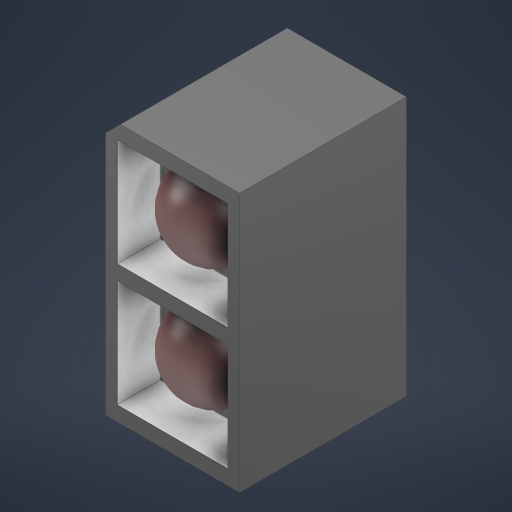
# Autodesk Inventor part: LBR127HLD
Saved by Autodesk Inventor 2023 (Build 270158000, 158)
## iProperties
Created: 2022-09-02
Part Number: LBR127HLD
Material: 一般
Document SubType Name: Modeling
Designer: neko2
Density: 1 g/cm^3
Appearance: 既定
Author: neko2
Autodesk Inventor part; units mm, degrees
ref_plane "YZ Plane" through (0, 0, 0) normal (1, 0, 0) x (0, 1, 0)
ref_plane "XZ Plane" through (0, 0, 0) normal (0, 1, 0) x (-1, 0, 0)
ref_plane "XY Plane" through (0, 0, 0) normal (0, 0, 1) x (1, 0, 0)
sketch "スケッチ1" plane through (0, 0, 0) normal (0, 0, 1) x (1, 0, 0)
  line L0 (0, 0) -> (4.5, 0)
  line L1 (4.5, 0) -> (4.5, 8.7)
  line L2 (4.5, 8.7) -> (0, 8.7)
  line L3 (0, 8.7) -> (0, 0)
  dimension "d0" = 4.5
  dimension "d1" = 8.7
  constraints: 8 end point, 3 perpendicular, 1 horizontal
  measures "d0" distance of L0.start L0.end
  measures "d1" distance of L0.end L1.end
extrude "押し出し1" add sketch "スケッチ1" against normal blind 5.6
chamfer "面取り1" distance 0.5 angle 45 1 edges at (0, 8.7, -2.8)
sketch "スケッチ2" plane through (0, 0, 0) normal (0, 0, 1) x (1, 0, 0)
  line L0 (0.4, 8.2) -> (4.1, 8.2)
  line L1 (4.1, 8.2) -> (4.1, 4.6)
  line L2 (4.1, 4.6) -> (0.4, 4.6)
  line L3 (0.4, 4.6) -> (0.4, 8.2)
  line L4 (0.4, 4.1) -> (4.1, 4.1)
  line L5 (4.1, 4.1) -> (4.1, 0.5)
  line L6 (4.1, 0.5) -> (0.4, 0.5)
  line L7 (0.4, 0.5) -> (0.4, 4.1)
  line L8 (0, 0) -> (4.5, 0) projected
  line L9 (4.5, 8.7) -> (0.5, 8.7) projected
  point P0 (2.25, 0)
  point P1 (2.25, 0.5)
  dimension "d7" = 3.7
  dimension "d8" = 3.6
  dimension "d9" = 3.6
  dimension "d10" = 0.5
  dimension "d11" = 0.5
  constraints: 16 end point, 4 parallel, 2 horizontal, 2 midpoint, 2 perpendicular, 2 point on line, 1 vertical alignment
  measures "d7" distance of L1.end L2.end
  measures "d8" distance of L0.end L1.end
  measures "d9" distance of L4.end L5.end
  measures "d10" distance between parallel lines of L9 L0
  measures "d11" distance between parallel lines of L8 L6
extrude "押し出し2" cut sketch "スケッチ2" against normal blind 1.45
sketch "スケッチ3" plane through (0, 0, -1.45) normal (0, 0, 1) x (1, 0, 0)
  line L0 (4.1, 4.6) -> (0.4, 4.6) projected
  line L1 (4.1, 8.2) -> (4.1, 4.6) projected
  line L2 (0.4, 8.2) -> (4.1, 8.2) projected
  line L3 (0.4, 4.6) -> (0.4, 8.2) projected
  line L4 (4.1, 0.5) -> (0.4, 0.5) projected
  line L5 (4.1, 4.1) -> (4.1, 0.5) projected
  line L6 (0.4, 4.1) -> (4.1, 4.1) projected
  line L7 (0.4, 0.5) -> (0.4, 4.1) projected
  circle A0 centre (2.25, 6.4) radius 1.45
  circle A1 centre (2.25, 2.3) radius 1.45
  line L8 (4.1, 4.1) -> (4.1, 0.5) projected
  line L9 (4.1, 8.2) -> (4.1, 4.6) projected
  line L10 (0.4, 8.2) -> (4.1, 8.2) projected
  line L11 (0.4, 4.1) -> (4.1, 4.1) projected
  point P0 (0, 0)
  point P1 (4.1, 2.3)
  point P2 (4.1, 6.4)
  point P3 (2.25, 8.2)
  point P4 (2.25, 4.1)
  dimension "d14" = 2.9
  dimension "d15" = 2.9
  constraints: 4 midpoint, 2 centre point, 2 horizontal alignment, 2 vertical alignment
  measures "d14" diameter of A0
  measures "d15" diameter of A1
extrude "押し出し3" add sketch "スケッチ3" along normal blind 1.45 contours A0 | A1
fillet "フィレット1" radius 1.45 2 edges at (0.8, 6.4, 0) (0.8, 2.3, 0)
